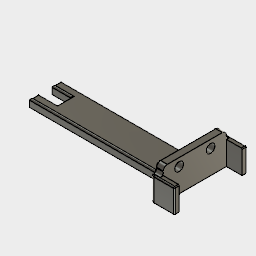
z-axis_centering_jig_v1 (Autodesk Fusion 360 design; units mm, degrees)
Autodesk Fusion 360 part; units mm, degrees
box "BoxPrimitive1" add length 40 width 5 height 20 placed x (0, 1, 0) y (-1, 0, 0) z (0, 0, 1) at (5, 0, 0) makes body 1
box "BoxPrimitive2" add length 3 width 15 height 15 placed x (0, -1, 0) y (1, 0, 0) z (0, 0, 1) at (0, 0, 0) separate body makes body 2
copy_body "CopyPasteBodies1" bodies 2 makes body 3
move_body "MoveBody1" bodies 3 to x (1, 0, 0) y (0, 1, 0) z (0, 0, 1) at (0, 43, 0)
cylinder "CylinderPrimitive1" add diameter 5.5 height -6 placed x (0, 0, -1) y (0, 1, 0) z (1, 0, 0) at (5, 0, 20) separate body makes body 4
move_body "MoveBody2" bodies 4 to x (1, 0, 0) y (0, 1, 0) z (0, 0, 1) at (1, 10, -5)
copy_body "CopyPasteBodies2" bodies 4 makes body 5
move_body "MoveBody3" bodies 5 to x (1, 0, 0) y (0, 1, 0) z (0, 0, 1) at (0, 20, 0)
box "BoxPrimitive3" add length 20 width 90 height 5 placed x (0, 1, 0) y (-1, 0, 0) z (0, 0, 1) at (90, 0, 0) separate body makes body 6
move_body "MoveBody4" bodies 6 to x (1, 0, 0) y (0, 1, 0) z (0, 0, 1) at (-90, 10, 0)
box "BoxPrimitive4" add length 8.5 width 26 height 6 placed x (0, 1, 0) y (-1, 0, 0) z (0, 0, 1) at (0, 0, 0) separate body makes body 7
move_body "MoveBody6" bodies 7 to x (1, 0, 0) y (0, 1, 0) z (0, 0, 1) at (0, 15.75, 0)
move_body "MoveBody7" bodies 7 to x (1, 0, 0) y (0, 1, 0) z (0, 0, 1) at (-78, 0, 0)
combine "Combine1" operation add target body 2 tool bodies 1 3 6
combine "Combine2" operation cut target body 2 tool bodies 4 5 7
fillet "Fillet1" radius 2 3 edges at (0, 30, 2.5) (0, 20, 5) (0, 10, 2.5) on bodies 2
fillet "Fillet2" radius 2 2 edges at (0, -3, 7.5) (0, 43, 7.5) on bodies 2
fillet "Fillet3" radius 2.5 2 edges at (2.5, 0, 20) (2.5, 40, 20) on bodies 2
fillet "Fillet4" radius 2 2 edges at (2.5, 0, 15) (2.5, 40, 15) on bodies 2
fillet "Fillet5" radius 0.75 13 edges at (8.5, 43, 15) (1, 42.7321, 15) (0.0638, 41.5012, 15.0632) (0, 40.2679, 16) (0, 40, 17.25) (0, 39.2678, 19.2678) (0, 20, 20) (0, 0.7322, 19.2678) (0, 0, 17.25) (0, -0.2679, 16) (0.0638, -1.5012, 15.0632) (1, -2.7321, 15) (8.5, -3, 15) on bodies 2
fillet "Fillet6" radius 0.5 2 edges at (0, 7.4361, 14.0056) (0, 27.4361, 14.0056) on bodies 2
fillet "Fillet7" radius 1 9 edges at (-84, 24.25, 5) (-78, 20, 5) (-84, 15.75, 5) (-90, 12.875, 5) (-90, 27.125, 5) (-0.5858, 30.5858, 5.5858) (-46, 30, 5) (-46, 10, 5) (-0.5858, 9.4142, 5.5858) on bodies 2
fillet "Fillet8" radius 0.5 6 edges at (15, -1.125, 15) (15, -2.7803, 14.7803) (15, -3, 7.125) (15, 41.125, 15) (15, 42.7803, 14.7803) (15, 43, 7.125) on bodies 2
